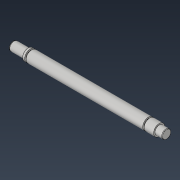
# Autodesk Inventor part: Dribblingwelle
Saved by Autodesk Inventor 2022.1 (Build 261234020, 234B)
## iProperties
Part Number: Dribblingwelle
Material: Aluminium 6061
Document SubType Name: Modeling
Designer: rYan
Density: 2.7 g/cm^3
Appearance: Aluminium - flach
Mass: 7.44424 g
Surface Area: 18.1797 cm^2
Volume: 2.75712 cm^3
Author: rYan
Autodesk Inventor part; units mm, degrees
ref_plane "YZ Plane" through (0, 0, 0) normal (1, 0, 0) x (0, 1, 0)
ref_plane "XZ Plane" through (0, 0, 0) normal (0, 1, 0) x (-1, 0, 0)
ref_plane "XY Plane" through (0, 0, 0) normal (0, 0, 1) x (1, 0, 0)
sketch "Skizze1" plane through (0, 0, 0) normal (0, 0, 1) x (1, 0, 0)
  line L0 (-44.3, 0) -> (44.3, 0)
  line L1 (44.3, 0) -> (44.3, 2.5)
  line L2 (44.3, 2.5) -> (40, 2.5)
  line L3 (40, 2.5) -> (40, 3.25)
  line L4 (33.7, 3.25) -> (-33.7, 3.25)
  line L5 (-35.7, 3.25) -> (-35.7, 2.5)
  line L6 (-35.7, 2.5) -> (-44.3, 2.5)
  line L7 (-44.3, 2.5) -> (-44.3, 0)
  line L8 (0, 3.9) -> (0, -0.65) projected
  line L9 (-39.8, 2.5) -> (-39.8, 0) construction
  line L10 (-33.7, 3.25) -> (-33.7, 2.5)
  line L11 (-33.7, 2.5) -> (-34.5, 2.5)
  line L12 (-34.5, 2.5) -> (-34.5, 3.25)
  line L13 (-34.5, 3.25) -> (-35.7, 3.25)
  line L14 (33.7, 3.25) -> (33.7, 2.5)
  line L15 (33.7, 2.5) -> (34.5, 2.5)
  line L16 (34.5, 2.5) -> (34.5, 3.25)
  line L17 (34.5, 3.25) -> (40, 3.25)
  point P0 (0, 0)
  dimension "d1" = 4.3
  dimension "d2" = 5
  dimension "d4" = 6.5
  dimension "d18" = 5
  dimension "d20" = 79.8
  dimension "d22" = 4.1
  dimension "d23" = 4.5
  dimension "d24" = 1.2
  dimension "d25" = 0.8
  dimension "d26" = 5
  constraints: 34 end point, 13 perpendicular, 3 collinear, 2 point on line, 2 vertical, 1 horizontal, 1 midpoint, 3 other
  measures "d1" distance of L1.end L2.end
  measures "d2" diameter of L2 L0
  measures "d4" diameter of L4 L0
  measures "d18" diameter of L6 L0
  measures "d20" distance between parallel lines of L3 L9
  measures "d22" distance between parallel lines of L5 L9
  measures "d23" distance between parallel lines of L7 L9
  measures "d24" distance between parallel lines of L5 L12
  measures "d25" distance of L10.end L11.end
  measures "d26" diameter of L11 L0
revolve "Umdrehung1" add sketch "Skizze1" angle 360 about axis through (-44.3, 0, 0) along (1, 0, 0)
chamfer "Fase2" distance 0.4 angle 15 1 edges at (-44.3, -2.5, 0) measured on face at (-41.4333, 2.4676, -0.401)
chamfer "Fase3" distance 0.4 angle 15 1 edges at (44.3, -2.5, 0) measured on face at (41.4333, 2.4676, -0.401)
